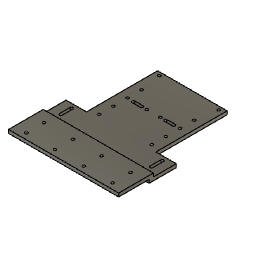
carBodyRearEnd v1 (Autodesk Fusion 360 design; units mm, degrees)
Autodesk Fusion 360 part; units mm, degrees
sketch "Sketch1" plane through (0, 0, 0) normal (0, 0, 1) x (1, 0, 0)
  line L0 (-45, 50) -> (37, 50)
  line L1 (37, 50) -> (37, 134)
  line L2 (37, 134) -> (-45, 134)
  line L3 (-45, 134) -> (-45, 50)
  line L4 (-69, 50) -> (61, 50)
  line L5 (61, 50) -> (61, -28)
  line L6 (61, -28) -> (-69, -28)
  line L7 (-69, -28) -> (-69, 50)
  line L8 (-30.5, -48) -> (22.5, -48)
  line L9 (22.5, -48) -> (22.5, -65)
  line L10 (22.5, -65) -> (-30.5, -65)
  line L11 (-30.5, -65) -> (-30.5, -48)
  line L12 (-60.5, -82) -> (52.5, -82)
  line L13 (52.5, -82) -> (52.5, -90)
  line L14 (52.5, -90) -> (-60.5, -90)
  line L15 (-60.5, -90) -> (-60.5, -82)
  line L16 (-30.5002, -118) -> (22.4998, -118)
  line L17 (22.4998, -118) -> (22.4998, -107)
  line L18 (22.4998, -107) -> (-30.5002, -107)
  line L19 (-30.5002, -107) -> (-30.5002, -118)
  line L20 (-44.0003, -127.9997) -> (35.9997, -127.9997)
  line L21 (35.9997, -127.9997) -> (35.9997, -132.9997)
  line L22 (35.9997, -132.9997) -> (-44.0003, -132.9997)
  line L23 (-44.0003, -132.9997) -> (-44.0003, -127.9997)
  circle A0 centre (-4.0003, -130.4997) radius 1.6
  circle A1 centre (1.9997, -130.4997) radius 1.6
  circle A2 centre (-10.0003, -130.4997) radius 1.6
  circle A3 centre (-18.0003, -130.4997) radius 1.6
  circle A4 centre (9.9997, -130.4997) radius 1.6
  line L24 (-10.0003, -128.8997) -> (-18.0003, -128.8997)
  line L25 (-10.0003, -132.0997) -> (-18.0003, -132.0997)
  line L26 (1.9997, -128.8997) -> (9.9997, -128.8997)
  line L27 (9.9997, -132.0997) -> (1.9997, -132.0997)
  line L28 (-45, 128.75) -> (-45, 134)
  line L29 (-45, 134) -> (-39.1, 134)
  line L30 (37, 134) -> (31, 134)
  line L31 (31, 134) -> (31, 130)
  line L32 (31, 130) -> (37, 130)
  line L33 (37, 130) -> (37, 134)
  line L34 (-45, 134) -> (-39, 134)
  line L35 (-39, 134) -> (-39, 130)
  line L36 (-39, 130) -> (-45, 130)
  line L37 (-45, 130) -> (-45, 134)
  circle A5 centre (-39, 130) radius 1.6
  circle A6 centre (31, 130) radius 1.6
  circle A7 centre (4.25, 87.9939) radius 1.6
  circle A8 centre (-11.75, 88.0061) radius 1.6
  line L38 (-11.75, 88.0061) -> (-17.75, 88.0107)
  circle A9 centre (-17.75, 88.0107) radius 1.6
  line L39 (4.25, 87.9939) -> (10.25, 87.9939)
  circle A10 centre (10.25, 87.9939) radius 1.6
  line L40 (10.25, 87.9939) -> (20.25, 87.9939)
  circle A11 centre (20.25, 87.9939) radius 1.6
  line L41 (-17.75, 88.0107) -> (-27.75, 88.0184)
  circle A12 centre (-27.75, 88.0184) radius 1.6
  line L42 (-27.7488, 89.6184) -> (-17.7488, 89.6107)
  line L43 (-27.7512, 86.4184) -> (-17.7512, 86.4107)
  line L44 (10.25, 89.5939) -> (20.25, 89.5939)
  line L45 (20.25, 86.3939) -> (10.25, 86.3939)
  line L46 (-69, 50) -> (-57.5, 50)
  line L47 (-57.5, 50) -> (-57.5, 45)
  line L48 (-57.5, 45) -> (-69, 45)
  line L49 (-69, 45) -> (-69, 50)
  circle A13 centre (-57.5, 45) radius 1.6
  line L50 (-57.5, 45) -> (-57.5, 32)
  circle A14 centre (-57.5, 32) radius 1.6
  line L51 (-55.9, 45.0023) -> (-55.9, 32)
  line L52 (-59.1, 45) -> (-59.1, 32)
  line L53 (61, 50) -> (49.5, 50)
  line L54 (49.5, 50) -> (49.5, 45)
  line L55 (49.5, 45) -> (61, 45)
  line L56 (61, 45) -> (61, 50)
  circle A15 centre (49.5, 45) radius 1.6
  line L57 (49.5, 45) -> (49.5, 32)
  circle A16 centre (49.5, 32) radius 1.6
  line L58 (51.1, 45) -> (51.1, 32)
  line L59 (47.9, 32) -> (47.9, 45)
  line L60 (-57.5, 45) -> (-57.5, -26)
  circle A17 centre (-57.5, -26) radius 1.6
  line L61 (49.5, 45) -> (49.5, -26)
  circle A18 centre (49.5, -26) radius 1.6
  circle A19 centre (-4, -51.9) radius 1.6
  circle A20 centre (33.037, -81.135) radius 1.6
  circle A21 centre (-41.033, -81.1414) radius 1.6
  line L62 (22.5, -48) -> (61, -28)
  line L63 (-30.5, -48) -> (-69, -28)
  line L64 (-60.5, -82) -> (-30.5, -65)
  line L65 (22.5, -65) -> (52.5, -82)
  line L66 (22.4998, -107) -> (52.5, -90)
  line L67 (-30.5002, -107) -> (-60.5, -90)
  line L68 (4.25, 87.9939) -> (-11.75, 88.0061)
  line L69 (-4, 134) -> (-3.75, 88)
  line L70 (-44.0003, -127.9997) -> (-30.5002, -118)
  line L71 (35.9997, -127.9997) -> (22.4998, -118)
  line L72 (-4.0003, -132.9997) -> (-4.0003, -138.9997)
  line L73 (-44.0003, -132.9997) -> (-4.0003, -138.9997)
  line L74 (-4.0003, -138.9997) -> (35.9997, -132.9997)
  line L75 (-4.0003, -130.4997) -> (1.9997, -130.4997)
  line L76 (-4.0003, -130.4997) -> (-10.0003, -130.4997)
  line L77 (-4, -65) -> (-4, -83)
  line L78 (-4, -83) -> (-4, -86)
  line L79 (-4, -86) -> (-56, -86)
  line L80 (-4, -86) -> (48, -86)
  circle A22 centre (48, -86) radius 1.1
  circle A23 centre (-56, -86) radius 1.1
  line L81 (20.25, 87.9939) -> (37, 87.9939)
  line L82 (-27.75, 88.0184) -> (-45, 88.0184)
  line L83 (37, 50) -> (24, 50)
  line L84 (24, 50) -> (24, 110)
  line L85 (24, 110) -> (37, 110)
  line L86 (37, 110) -> (37, 50)
  line L87 (-45, 50) -> (-32, 50)
  line L88 (-32, 50) -> (-32, 110)
  line L89 (-32, 110) -> (-45, 110)
  line L90 (-45, 110) -> (-45, 50)
  line L91 (37, 110) -> (31, 110)
  line L92 (31, 110) -> (31, 50)
  line L93 (31, 50) -> (37, 50)
  line L94 (37, 50) -> (37, 110)
  line L95 (-45, 110) -> (-39, 110)
  line L96 (-39, 110) -> (-39, 50)
  line L97 (-39, 50) -> (-45, 50)
  line L98 (-45, 50) -> (-45, 110)
  line L99 (24, 110) -> (27, 110)
  line L100 (27, 110) -> (27, 105)
  line L101 (27, 105) -> (24, 105)
  line L102 (24, 105) -> (24, 110)
  circle A24 centre (27, 105) radius 1.6
  circle A25 centre (27, 88.3333) radius 1.6
  circle A26 centre (27, 71.6667) radius 1.6
  circle A27 centre (27, 55) radius 1.6
  line L103 (-32, 110) -> (-35, 110)
  line L104 (-35, 110) -> (-35, 105)
  line L105 (-35, 105) -> (-32, 105)
  line L106 (-32, 105) -> (-32, 110)
  circle A28 centre (-35, 105) radius 1.6
  circle A29 centre (-35, 88.3333) radius 1.6
  circle A30 centre (-35, 71.6667) radius 1.6
  circle A31 centre (-35, 55) radius 1.6
  line L107 (-69, -28) -> (-49.75, -28)
  line L108 (-49.75, -28) -> (-49.75, -18)
  line L109 (-49.75, -18) -> (-69, -18)
  line L110 (-69, -18) -> (-69, -28)
  line L111 (-69, -18) -> (61, -18)
  line L112 (61, -18) -> (61, 17)
  line L113 (61, 17) -> (-69, 17)
  line L114 (-69, 17) -> (-69, -18)
  line L115 (-69, 17) -> (-55, 17)
  line L116 (-55, 17) -> (-55, 10)
  line L117 (-55, 10) -> (-69, 10)
  line L118 (-69, 10) -> (-69, 17)
  line L119 (61, 17) -> (47, 17)
  line L120 (47, 17) -> (47, 10)
  line L121 (47, 10) -> (61, 10)
  line L122 (61, 10) -> (61, 17)
  circle A32 centre (-55, 10) radius 1.6
  circle A33 centre (-21, 10) radius 1.6
  circle A34 centre (13, 10) radius 1.6
  circle A35 centre (47, 10) radius 1.6
  circle A36 centre (-55, -11) radius 1.6
  circle A37 centre (-21, -11) radius 1.6
  circle A38 centre (13, -11) radius 1.6
  circle A39 centre (47, -11) radius 1.6
  line L123 (-69, 17) -> (61, 17)
  line L124 (61, 17) -> (61, 18)
  line L125 (61, 18) -> (-69, 18)
  line L126 (-69, 18) -> (-69, 17)
  line L127 (61, 18) -> (-69, 18)
  line L128 (-69, 18) -> (-69, 23)
  line L129 (-69, 23) -> (61, 23)
  line L130 (61, 23) -> (61, 18)
  circle A40 centre (18.0038, -78.6409) radius 1.6
  circle A41 centre (18.0038, -78.6409) radius 5
  circle A42 centre (-25.9962, -78.6409) radius 5
  circle A43 centre (-25.9962, -78.6409) radius 1.6
  dimension "d1" = 82
  dimension "d2" = 84
  dimension "d3" = 78
  dimension "d4" = 130
  dimension "d6" = 17
  dimension "d11" = 113
  dimension "d12" = 8
  dimension "d15" = 11
  dimension "d16" = 53
  dimension "d20" = 80
  dimension "d21" = 5
  dimension "d25" = 3.2
  dimension "d29" = 3.2
  dimension "d31" = 3.2
  dimension "d32" = 3.2
  dimension "d35" = 3.2
  dimension "d38" = 6
  dimension "d39" = 4
  dimension "d42" = 6
  dimension "d43" = 4
  dimension "d44" = 3.2
  dimension "d45" = 3.2
  dimension "d53" = 3.2
  dimension "d54" = 3.2
  dimension "d55" = 6
  dimension "d56" = 3.2
  dimension "d58" = 6
  dimension "d59" = 3.2
  dimension "d60" = 10
  dimension "d61" = 3.2
  dimension "d62" = 10
  dimension "d63" = 3.2
  dimension "d64" = 11.5
  dimension "d65" = 3.2
  dimension "d66" = 13
  dimension "d67" = 3.2
  dimension "d68" = 11.5
  dimension "d69" = 5
  dimension "d70" = 5
  dimension "d71" = 3.2
  dimension "d72" = 13
  dimension "d73" = 3.2
  dimension "d74" = 71
  dimension "d75" = 3.2
  dimension "d77" = 71
  dimension "d78" = 3.2
  dimension "d80" = 3.2
  dimension "d83" = 3.2
  dimension "d84" = 3.2
  dimension "d90" = 53
  dimension "d92" = 46
  dimension "d93" = 16
  dimension "d95" = 6
  dimension "d99" = 6
  dimension "d100" = 6
  dimension "d101" = 8
  dimension "d102" = 8
  dimension "d108" = 52
  dimension "d109" = 52
  dimension "d110" = 2.2
  dimension "d111" = 2.2
  dimension "d112" = 13
  dimension "d113" = 60
  dimension "d114" = 13
  dimension "d115" = 60
  dimension "d116" = 60
  dimension "d117" = 6
  dimension "d118" = 60
  dimension "d119" = 3
  dimension "d120" = 5
  dimension "d121" = 3.2
  dimension "d124" = 0
  dimension "d125" = -50
  dimension "d126" = 3
  dimension "d127" = 5
  dimension "d128" = 3.2
  dimension "d131" = 0
  dimension "d132" = -50
  dimension "d133" = 10
  dimension "d134" = 35
  dimension "d135" = 14
  dimension "d136" = 7
  dimension "d137" = 14
  dimension "d138" = 7
  dimension "d139" = 3.2
  dimension "d142" = 102
  dimension "d143" = -21
  dimension "d144" = 1
  dimension "d145" = 130
  dimension "d146" = 5
  dimension "d154" = 3.2
  dimension "d155" = 10
  dimension "d156" = 3.2
  dimension "d157" = 10
  constraint horizontal L0
  constraint vertical L1
  constraint horizontal L2
  constraint vertical L3
  constraint horizontal L4
  constraint vertical L5
  constraint horizontal L6
  constraint vertical L7
  constraint horizontal L8
  constraint vertical L9
  constraint horizontal L10
  constraint vertical L11
  constraint horizontal L12
  constraint vertical L13
  constraint horizontal L14
  constraint vertical L15
  constraint horizontal L16
  constraint vertical L17
  constraint horizontal L18
  constraint vertical L19
  constraint vertical L21
  constraint horizontal L22
  constraint vertical L23
  constraint coincident A2 L24.start
  constraint coincident A3 L24.end
  constraint tangent A3 L24
  constraint coincident A2 L25.start
  constraint coincident A3 L25.end
  constraint tangent A3 L25
  constraint coincident A1 L26.start
  constraint coincident A4 L26.end
  constraint tangent A4 L26
  constraint coincident A4 L27.start
  constraint coincident A1 L27.end
  constraint tangent A1 L27
  constraint vertical L28
  constraint horizontal L29
  constraint horizontal L30
  constraint vertical L31
  constraint horizontal L32
  constraint vertical L33
  constraint horizontal L34
  constraint vertical L35
  constraint horizontal L36
  constraint vertical L37
  constraint coincident L35.end L36.start
  constraint coincident L31.end L32.start
  constraint coincident A8.centre L38.start
  constraint coincident L38.end A9.centre
  constraint coincident A7.centre L39.start
  constraint coincident L39.end A10.centre
  constraint coincident L40.end A11.centre
  constraint coincident L41.end A12.centre
  constraint coincident A12 L42.start
  constraint coincident A9 L42.end
  constraint tangent A9 L42
  constraint coincident A12 L43.start
  constraint coincident A9 L43.end
  constraint tangent A9 L43
  constraint coincident A10 L44.start
  constraint coincident A11 L44.end
  constraint tangent A11 L44
  constraint coincident A11 L45.start
  constraint coincident A10 L45.end
  constraint tangent A10 L45
  constraint horizontal L46
  constraint vertical L47
  constraint horizontal L48
  constraint vertical L49
  constraint coincident L47.end L48.start
  constraint perpendicular L48 L50
  constraint coincident L50.end A14.centre
  constraint coincident A13 L51.start
  constraint coincident A14 L51.end
  constraint tangent A14 L51
  constraint parallel L47 L51
  constraint coincident A13 L52.start
  constraint coincident L48 L52.start
  constraint coincident A14 L52.end
  constraint tangent A14 L52
  constraint horizontal L53
  constraint vertical L54
  constraint horizontal L55
  constraint vertical L56
  constraint coincident L54.end L55.start
  constraint perpendicular L55 L57
  constraint coincident L57.end A16.centre
  constraint coincident A15 L58.start
  constraint coincident L55 L58.start
  constraint coincident A16 L58.end
  constraint tangent A16 L58
  constraint coincident A16 L59.start
  constraint coincident A15 L59.end
  constraint tangent A15 L59
  constraint parallel L50 L60
  constraint coincident L60.end A17.centre
  constraint perpendicular L55 L61
  constraint coincident L61.end A18.centre
  constraint midpoint L2 L69.start
  constraint midpoint L68 L69.end
  constraint tangent A10 L44
  constraint tangent A11 L45
  constraint tangent A12 L42
  constraint tangent A12 L43
  constraint midpoint L22 L72.start
  constraint perpendicular L22 L72
  constraint coincident A0.centre L75.start
  constraint coincident A1.centre L75.end
  constraint coincident A2.centre L76.end
  constraint tangent A2 L24
  constraint tangent A2 L25
  constraint tangent A1 L26
  constraint tangent A4 L27
  constraint midpoint L10 L77.start
  constraint perpendicular L78 L79
  constraint perpendicular L78 L80
  constraint coincident L80.end A22.centre
  constraint coincident L79.end A23.centre
  constraint coincident L1 L81.end
  constraint perpendicular L1 L81
  constraint coincident L3 L82.end
  constraint perpendicular L3 L82
  constraint horizontal L83
  constraint vertical L84
  constraint horizontal L85
  constraint vertical L86
  constraint horizontal L87
  constraint vertical L88
  constraint horizontal L89
  constraint vertical L90
  constraint horizontal L91
  constraint vertical L92
  constraint horizontal L93
  constraint vertical L94
  constraint horizontal L95
  constraint vertical L96
  constraint horizontal L97
  constraint vertical L98
  constraint horizontal L99
  constraint vertical L100
  constraint horizontal L101
  constraint vertical L102
  constraint coincident L100.end L101.start
  constraint horizontal L103
  constraint vertical L104
  constraint horizontal L105
  constraint vertical L106
  constraint coincident L104.end L105.start
  constraint horizontal L107
  constraint vertical L108
  constraint horizontal L109
  constraint vertical L110
  constraint horizontal L111
  constraint vertical L112
  constraint horizontal L113
  constraint vertical L114
  constraint horizontal L115
  constraint vertical L116
  constraint horizontal L117
  constraint vertical L118
  constraint horizontal L119
  constraint vertical L120
  constraint horizontal L121
  constraint vertical L122
  constraint coincident L116.end L117.start
  constraint horizontal L123
  constraint vertical L124
  constraint horizontal L125
  constraint vertical L126
  constraint coincident L5 L124.end
  constraint horizontal L127
  constraint vertical L128
  constraint horizontal L129
  constraint vertical L130
  constraint concentric A40 A41
  constraint concentric A42 A43
  measures "d1" distance of L1.end L2.end
  measures "d2" distance of L0.start L2.end
  measures "d3" distance of L4.end L5.end
  measures "d4" distance of L5.end L6.end
  measures "d6" distance of L8.start L10.end
  measures "d11" distance of L12.start L12.end
  measures "d12" distance of L12.start L14.end
  measures "d15" distance of L16.start L18.end
  measures "d16" distance of L17.end L18.end
  measures "d20" distance of L20.start L20.end
  measures "d21" distance of L20.start L22.end
  measures "d25" diameter of A0
  measures "d29" diameter of A1
  measures "d31" diameter of A2
  measures "d32" diameter of A3
  measures "d35" diameter of A4
  measures "d38" distance of L1.end L30.end
  measures "d39" distance of L1.end L32.end
  measures "d42" distance of L2.end L34.end
  measures "d43" distance of L2.end L36.end
  measures "d44" diameter of A5
  measures "d45" diameter of A6
  measures "d53" diameter of A7
  measures "d54" diameter of A8
  measures "d55" distance of A8.centre L38.end
  measures "d56" diameter of A9
  measures "d58" distance of A7.centre L39.end
  measures "d59" diameter of A10
  measures "d60" distance of L39.end L40.end
  measures "d61" diameter of A11
  measures "d62" distance of L38.end L41.end
  measures "d63" diameter of A12
  measures "d64" distance of L4.start L46.end
  measures "d65" diameter of A13
  measures "d66" distance of L47.end L50.end
  measures "d67" diameter of A14
  measures "d68" distance of L4.end L53.end
  measures "d69" distance of L4.end L55.end
  measures "d70" distance of L4.start L48.end
  measures "d71" diameter of A15
  measures "d72" distance of L54.end L57.end
  measures "d73" diameter of A16
  measures "d74" distance of L47.end L60.end
  measures "d75" diameter of A17
  measures "d77" distance of L54.end L61.end
  measures "d78" diameter of A18
  measures "d80" diameter of A19
  measures "d83" diameter of A20
  measures "d84" diameter of A21
  measures "d90" distance of L8.start L8.end
  measures "d92" vertical distance of L69.start L69.end
  measures "d93" horizontal distance of A7.centre A8.centre
  measures "d95" distance of L72.start L72.end
  measures "d99" distance of A0.centre A1.centre
  measures "d100" distance of A0.centre A2.centre
  measures "d101" distance of L24.start L24.end
  measures "d102" distance of L26.start L26.end
  measures "d108" distance of L78.end L79.end
  measures "d109" distance of L78.end L80.end
  measures "d110" diameter of A22
  measures "d111" diameter of A23
  measures "d112" distance of L0.end L83.end
  measures "d113" distance of L0.end L85.end
  measures "d114" distance of L0.start L87.end
  measures "d115" distance of L0.start L89.end
  measures "d116" distance of L85.end L0.end
  measures "d117" distance of L89.end L95.end
  measures "d118" distance of L89.end L0.start
  measures "d119" distance of L84.end L99.end
  measures "d120" distance of L84.end L101.end
  measures "d121" diameter of A24
  measures "d126" distance of L88.end L103.end
  measures "d127" distance of L88.end L105.end
  measures "d128" diameter of A28
  measures "d133" distance of L6.end L109.end
  measures "d134" distance of L109.end L113.end
  measures "d135" distance of L113.end L115.end
  measures "d136" distance of L113.end L117.end
  measures "d137" distance of L112.end L119.end
  measures "d138" distance of L112.end L121.end
  measures "d139" diameter of A32
  measures "d144" distance of L113.end L125.end
  measures "d145" distance of L124.end L125.end
  measures "d146" distance of L124.end L129.end
  measures "d154" diameter of A40
  measures "d155" diameter of A41
  measures "d156" diameter of A43
  measures "d157" diameter of A42
extrude "Extrude2" add sketch "Sketch1" along normal blind 4 contours L0 L3 L4 L82 L87 L90 L96 L97 L98 | L0 L4 L47 A13 A14 L51 L54 A15 A16 L59 L60 L61 L83 L87 L93 L97 L129 | L0 L4 L82 L87 L88 L96 A29 | L3 L82 L89 L90 L95 L96 L98 | L4 L7 L46 L47 L48 L49 A13 | L0 L4 A7 A8 L38 A9 L39 A10 A11 A12 L43 L45 L68 L81 L82 L84 L88 | L82 L88 L89 L96 L104 L105 A28 A29 | L2 L3 L28 L35 L36 A5 A8 L38 A9 A12 L42 L68 L69 L82 L88 L89 L95 L103 L106 | L0 L4 L81 L83 L84 L92 A25 | L7 L48 A14 L52 L60 L129 | L0 L1 L4 L81 L83 L86 L92 L93 L94 | L81 L84 L85 L92 L100 L101 A24 A25 | L1 L2 L31 L32 A6 A7 L39 A10 A11 L44 L68 L69 L81 L84 L85 L91 L99 L102 | L88 L89 L103 L104 L105 L106 A28 | L2 L3 L28 L29 L34 L35 L36 L37 A5 | L7 L60 L125 L127 L128 L129 | L1 L81 L85 L86 L91 L92 L94 | L84 L85 L99 L100 L101 L102 A24 | L60 L61 L125 L127 L129 | L4 L5 L53 L54 L55 L56 A15 | L5 L61 L125 L127 L129 L130 | L5 L55 A16 L58 L61 L129 | L1 L2 L30 L31 L32 L33 A6
extrude "Extrude3" add sketch "Sketch1" along normal blind 4 from surface at 4 contours L7 L60 L125 L127 L128 L129 | L7 L60 L113 L115 L123 L125 L126 L127 | L60 L61 L125 L127 L129 | L7 L60 L113 L114 L115 L117 L118 L123 | L60 L61 L113 L115 L119 L123 L125 L127 | L5 L61 L125 L127 L129 L130 | L7 L60 L109 L111 L114 L117 | L60 L113 L115 L116 L117 A32 L123 | L5 L61 L113 L119 L123 L124 L125 L127 | L60 L61 L109 L111 L113 L116 L117 L120 L121 A32 A35 L123 | L5 L61 L112 L113 L119 L121 L122 L123 | L61 L113 L119 L120 L121 A35 L123 | L5 L61 L111 L112 L121
extrude "Extrude4" [suppressed]
equation "d108 = ( 104 / 2 ) * 1 mm"
equation "d109 = ( 104 / 2 ) * 1 mm"
named bodies: "CarBodyRearEnd", "CarBodyFrontEnd"
